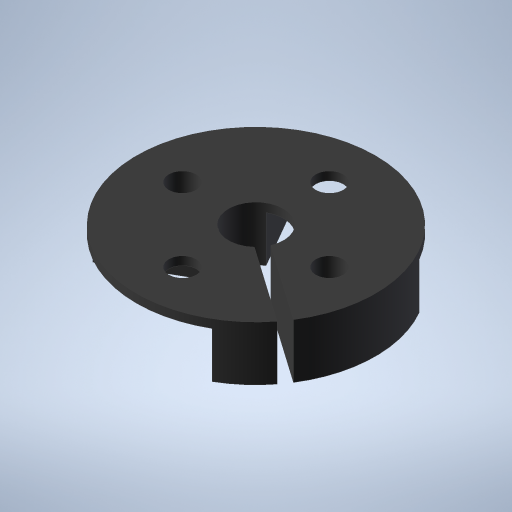
# Autodesk Inventor part: tab3
Saved by Autodesk Inventor 2024 (Build 280153000, 153)
## iProperties
Created: 2023-04-25
Part Number: tab3
Material: Generic
Document SubType Name: Modeling
Designer: Fujitsu
Density: 1 g/cm^3
Appearance: Default
Author: Fujitsu
Autodesk Inventor part; units mm, degrees
ref_plane "YZ Plane" through (0, 0, 0) normal (1, 0, 0) x (0, 1, 0)
ref_plane "XZ Plane" through (0, 0, 0) normal (0, 1, 0) x (-1, 0, 0)
ref_plane "XY Plane" through (0, 0, 0) normal (0, 0, 1) x (1, 0, 0)
sketch "Sketch1" plane through (0, 0, 0) normal (0, 1, 0) x (-1, 0, 0)
  circle A0 centre (0, 0) radius 3.81
  circle A1 centre (0, 0) radius 16.51
  line L0 (0, 0) -> (10.16, 0)
  line L1 (0, 0) -> (-10.16, 0)
  circle A2 centre (10.16, 0) radius 1.524
  circle A3 centre (-10.16, 0) radius 1.524
  circle A4 centre (0, 0) radius 5.0292
  circle A5 centre (0, 0) radius 15.2908
  line L2 (0, 0) -> (0, 10.16)
  circle A6 centre (0, 10.16) radius 2.3812
  line L3 (0, 0) -> (2.5146, 4.3554)
  line L4 (0, 0) -> (5.0292, 0) construction
  line L5 (2.5146, 4.3554) -> (7.6454, 13.2422)
  line L6 (0, 0) -> (-2.5146, 4.3554)
  line L7 (-2.5146, 4.3554) -> (-7.6454, 13.2422)
  line L8 (0, 0) -> (2.5146, -4.3554)
  line L9 (2.5146, -4.3554) -> (7.6454, -13.2422)
  line L10 (0, 0) -> (-2.5146, -4.3554)
  line L11 (-2.5146, -4.3554) -> (-7.6454, -13.2422)
  line L12 (0.4064, 16.8443) -> (-0.4064, 16.8443)
  line L13 (-0.4064, 16.8443) -> (-0.4064, 15.0672)
  line L14 (-0.4064, 15.0672) -> (0.4064, 15.0672)
  line L15 (0.4064, 15.0672) -> (0.4064, 16.8443)
  line L16 (0.4064, 16.8443) -> (-0.4064, 15.0672) construction
  line L17 (-0.4064, 16.8443) -> (0.4064, 15.0672) construction
  line L18 (0.4064, -15.0362) -> (-0.4064, -15.0362)
  line L19 (-0.4064, -15.0362) -> (-0.4064, -16.8142)
  line L20 (-0.4064, -16.8142) -> (0.4064, -16.8142)
  line L21 (0.4064, -16.8142) -> (0.4064, -15.0362)
  line L22 (0.4064, -15.0362) -> (-0.4064, -16.8142) construction
  line L23 (-0.4064, -15.0362) -> (0.4064, -16.8142) construction
  circle A7 centre (0, 10.16) radius 1.524
  line L24 (0, 0) -> (0, -10.16)
  circle A8 centre (0, -10.16) radius 1.524
  circle A9 centre (0, 0) radius 0.7937
  line L25 (0, 0) -> (-13.5242, 9.4697)
  line L26 (0, 0) -> (16.51, 0) construction
  line L27 (-13.9904, 8.8039) -> (-0.408, -0.7066)
  line L28 (-13.058, 10.1356) -> (0.2563, 0.8128)
  line L29 (16.49, 0.8128) -> (16.51, 0.8128)
  line L30 (16.49, -0.8128) -> (16.51, -0.8128)
  line L31 (0, 0) -> (-0.408, -0.7066)
  line L32 (0.2563, 0.8128) -> (0.408, 0.7066)
  line L33 (0, 0) -> (0.408, 0.7066)
  line L34 (-13.058, 10.1356) -> (-13.9904, 8.8039)
  line L35 (0.408, 0.7066) -> (-0.408, -0.7066)
  line L36 (-7.6454, 13.2422) -> (-8.255, 14.2981)
  line L37 (7.6454, 13.2422) -> (8.255, 14.2981)
  line L38 (-7.6454, -13.2422) -> (-8.255, -14.2981)
  line L39 (7.6454, -13.2422) -> (8.255, -14.2981)
  line L40 (0, 0) -> (13.2422, 7.6454)
  line L41 (13.2422, 7.6454) -> (14.2981, 8.255)
  line L42 (0, 0) -> (-13.2422, -7.6454)
  line L43 (-13.2422, -7.6454) -> (-14.2981, -8.255)
  point P0 (0, 15.9557)
  point P1 (0, -15.9252)
  point P2 (-13.974, 8.7925)
  point P3 (-1.4171, 0)
  point P4 (-0.7937, 0)
  point P5 (-0.3969, 0.6874)
  point P6 (-0.9616, 1.6656)
  point P7 (-13.0416, 10.1241)
  point P8 (1.905, 3.2996)
  point P9 (-1.905, 3.2996)
  point P10 (1.905, -3.2996)
  point P11 (-1.905, -3.2996)
  point P12 (4.3554, 2.5146)
  point P13 (-4.3554, -2.5146)
  point P14 (3.2996, 1.905)
  point P15 (-3.2996, -1.905)
  dimension "d1" = 33.02
  dimension "d0" = 7.62
  dimension "d2" = 10.16
  dimension "d3" = 10.16
  dimension "d4" = 3.048
  dimension "d5" = 3.048
  dimension "d8" = 10.0584
  dimension "d9" = 30.5816
  dimension "d10" = 10.16
  dimension "d11" = 4.7625
  dimension "d12" = 60
  dimension "d17" = 0.8128
  dimension "d18" = 0.8128
  dimension "d19" = 1.778
  dimension "d24" = 3.048
  dimension "d25" = 10.16
  dimension "d26" = 3.048
  dimension "d41" = 1.5875
  dimension "d42" = 145
  dimension "d43" = 0.8128
  dimension "d44" = 0.8128
  constraints: 88 end point, 10 coincident, 10 point on circle, 9 centre point, 6 horizontal, 6 point on line, 4 midpoint, 4 parallel, 4 perpendicular, 2 collinear, 2 equal length, 1 vertical, 11 other
  measures "d0" diameter of A0
  measures "d2" distance of L0.start L0.end
  measures "d3" distance of L0.start L1.end
  measures "d4" diameter of A2
  measures "d5" diameter of A3
  measures "d8" diameter of A4
  measures "d9" diameter of A5
  measures "d10" distance of L2.start L2.end
  measures "d11" diameter of A6
  measures "d12" angle of L4 L3
  measures "d17" distance of L14.end L13.end
  measures "d18" distance of L20.end L19.end
  measures "d19" distance of L19.end L18.end
  measures "d24" diameter of A7
  measures "d25" distance of L2.start L24.end
  measures "d26" diameter of A8
  measures "d41" diameter of A9
  measures "d42" angle of L26 L25
  measures "d43" distance between parallel lines of L25 L27
  measures "d44" distance between parallel lines of L25 L28
extrude "Extrusion1" add sketch "Sketch1" along normal blind 7.5184 contours L0 A4 L8 A0 | A0 L40 A4 L0 | A0 L3 A4 L40 | L8 A4 L24 A0 | A2 | A4 L40 A5 L9 | A0 L2 A4 L3 | A4 L5 A5 L40 | L24 A4 L10 A0 | A8 | L9 A5 L21 L18 L19 L11 A4 | A0 L6 A4 L2 | A7 | A6 | A4 L7 A5 L13 L14 L15 L5 | L41 A1 L39 A5 | A5 L37 A1 L41 | L10 A4 L42 A0 | L39 A1 L21 A5 | A0 L28 A4 L6 | A5 L15 A1 L37 | L42 A4 L1 A0 | L11 A5 L42 A4 | L21 A1 L19 A5 | A5 L19 L18 L21 | L25 A4 L28 A0 | A0 L27 A4 L25 | A4 L28 A5 L7 | L15 L14 L13 A5 | A5 L13 A1 L15 | L1 A4 L27 A0 | A3 | L42 A5 L27 A4 | L38 A1 L43 A5 | A5 L19 A1 L38 | L25 A5 L28 A4 | A4 L27 A5 L25 | L36 A1 L13 A5 | A5 L28 A1 L36 | L43 A1 L27 A5 | L25 A1 L28 A5 | A5 L27 A1 L25
extrude "Extrusion2" cut sketch "Sketch1" along normal blind 6.35 contours A0 L3 A4 L40 | A0 L2 A4 L3 | A4 L5 A5 L40 | A0 L6 A4 L2 | A7 | A6 | A4 L7 A5 L13 L14 L15 L5 | A5 L37 A1 L41 | A5 L15 A1 L37 | L15 L14 L13 A5 | A5 L13 A1 L15 | L36 A1 L13 A5
extrude "Extrusion3" cut sketch "Sketch1" along normal blind 6.35 contours L8 A4 L24 A0 | L24 A4 L10 A0 | A8 | L9 A5 L21 L18 L19 L11 A4 | L10 A4 L42 A0 | L39 A1 L21 A5 | L11 A5 L42 A4 | L21 A1 L19 A5 | A5 L19 L18 L21 | L38 A1 L43 A5 | A5 L19 A1 L38
extrude "Extrusion6" cut sketch "Sketch1" along normal blind 7.5184 contours L1 L27 A0 L25 A9 | A9 L25 A0 L28 L6 | L25 A4 L28 A0 | A0 L27 A4 L25 | L25 A5 L28 A4 | A4 L27 A5 L25 | L25 A1 L28 A5 | A5 L27 A1 L25
hole "Hole3" at (10.16, 0, 0) direction (0, 1, 0) diameter 3.81 end through all clearance for "Flat Head Machine Screw (82)" size "#6" standard "Ansi Unified Screw Threads"
hole "Hole4" at (-10.16, 0, 0) direction (0, 1, 0) diameter 3.81 end through all clearance for "Flat Head Machine Screw (82)" size "#6" standard "Ansi Unified Screw Threads"
hole "Hole5" at (0, 0, -10.16) direction (0, 1, 0) diameter 3.81 end through all clearance for "Flat Head Machine Screw (82)" size "#6" standard "Ansi Unified Screw Threads"
hole "Hole6" at (0, 0, 10.16) direction (0, 1, 0) diameter 3.81 end through all clearance for "Flat Head Machine Screw (82)" size "#6" standard "Ansi Unified Screw Threads"
body "Solid1"
